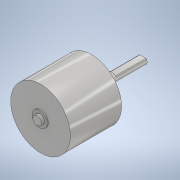
# Autodesk Inventor part: Part5
Saved by Autodesk Inventor 2021 (Build 250183000, 183)
## iProperties
Created: 2020-06-30
Part Number: Part5
Material: Genérico
Document SubType Name: Modeling
Designer: IVAN
Density: 1 g/cm^3
Appearance: Aluminum - Polished
Author: IVAN
Autodesk Inventor part; units mm, degrees
ref_plane "YZ Plane" through (0, 0, 0) normal (1, 0, 0) x (0, 1, 0)
ref_plane "XZ Plane" through (0, 0, 0) normal (0, 1, 0) x (-1, 0, 0)
ref_plane "XY Plane" through (0, 0, 0) normal (0, 0, 1) x (1, 0, 0)
sketch "Sketch1" plane through (0, 0, 0) normal (0, 1, 0) x (-1, 0, 0)
  circle A0 centre (0, 0) radius 17.5
  dimension "d0" = 35
  constraints: 1 centre point, 1 coincident
  measures "d0" diameter of A0
extrude "Extrusion1" add sketch "Sketch1" along normal blind 30
sketch "Sketch2" plane through (0, 0, 0) normal (0, -1, 0) x (1, 0, 0)
  circle A0 centre (0, 0) radius 2.5
  dimension "d3" = 5
  constraints: 1 centre point, 1 coincident
  measures "d3" diameter of A0
extrude "Extrusion2" add sketch "Sketch2" along normal blind 2
sketch "Sketch3" plane through (0, 30, 0) normal (0, 1, 0) x (1, 0, 0)
  circle A0 centre (0, 0) radius 2.5
  dimension "d6" = 5
  constraints: 1 centre point, 1 coincident
  measures "d6" diameter of A0
extrude "Extrusion3" add sketch "Sketch3" along normal blind 30
sketch "Sketch4" plane through (0, 30, 0) normal (0, 1, 0) x (1, 0, 0)
  circle A0 centre (0, 0) radius 4.5
  circle A1 centre (0, 0) radius 2.75
  dimension "d9" = 9
  dimension "d12" = 5.5
  constraints: 2 centre point, 2 coincident
  measures "d9" diameter of A0
  measures "d12" diameter of A1
extrude "Extrusion5" add sketch "Sketch4" along normal blind 3
sketch "Sketch5" plane through (0, 0, 0) normal (0, -1, 0) x (1, 0, 0)
  circle A0 centre (0, 0) radius 2.75
  circle A1 centre (0, 0) radius 4.5
  dimension "d15" = 5.5
  dimension "d16" = 9
  constraints: 2 centre point, 2 coincident
  measures "d15" diameter of A0
  measures "d16" diameter of A1
extrude "Extrusion6" add sketch "Sketch5" along normal blind 0.5
sketch "Sketch6" plane through (0, 60, 0) normal (0, 1, 0) x (1, 0, 0)
  line L0 (2.243, -1.5) -> (-2.3112, -1.5)
  circle A0 centre (0, 0) radius 2.75 projected
  circle A1 centre (0, 0) radius 2.5 projected
  circle A2 centre (0, 0) radius 2.5 projected
  line L1 (2, -1.5) -> (-2, -1.5)
  dimension "d19" = 1.5
  constraints: 4 end point, 2 point on circle, 2 point on line, 1 horizontal
  measures "d19" distance from line of point (0, 0) L0
extrude "Extrusion7" cut sketch "Sketch6" against normal blind 18 contours A1 L0 picked at (-0.534, -1.6398)
fillet "Fillet1" radius 0.5 2 edges at (2, 51, 1.5) (-2, 51, 1.5)
body "Solid1"
